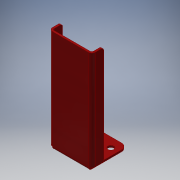
# Autodesk Inventor part: Supporto pistone pinza
Saved by Autodesk Inventor 2018 (Build 220112000, 112)
## iProperties
Created: 2020-05-29
Part Number: Supporto pistone pinza
Material: Generico
Document SubType Name: Lamiera
Designer: Francesco
Density: 1 g/cm^3
Sheet Metal Rule: Default_mm
Appearance: Rosso
Author: Francesco
Autodesk Inventor part; units mm, degrees
ref_plane "YZ Plane" through (0, 0, 0) normal (1, 0, 0) x (0, 1, 0)
ref_plane "XZ Plane" through (0, 0, 0) normal (0, 1, 0) x (-1, 0, 0)
ref_plane "XY Plane" through (0, 0, 0) normal (0, 0, 1) x (1, 0, 0)
sketch "Schizzo1" plane through (0, 0, 0) normal (0, 0, 1) x (1, 0, 0)
  line L0 (-15, 15) -> (15, 15)
  line L1 (15, 15) -> (15, -15)
  line L2 (15, -15) -> (-15, -15)
  line L3 (-15, -15) -> (-15, 15)
  line L4 (-15, 15) -> (15, -15) construction
  line L5 (15, 15) -> (-15, -15) construction
  point P0 (0, 0)
  dimension "d0" = 30
  dimension "d1" = 30
  measures "d0" distance of L1.end L2.end
  measures "d1" distance of L0.end L1.end
extrude "Piano1" add sketch "Schizzo1" along normal blind 1.5
sketch "Schizzo2" plane through (15, -16.5, 3) normal (0, -1, 0) x (1, 0, 0)
  line L0 (-30, 0) -> (0, 0)
  line L1 (0, 0) -> (0, 83.5)
  line L2 (0, 83.5) -> (-30, 83.5)
  line L3 (-30, 83.5) -> (-30, 0)
  constraints: 6 end point, 1 horizontal, 1 perpendicular, 1 vertical
edge flange "Flangia1" height 86.5 angle 90 thickness 1.5 bend radius 1.5 thickness toward (0, -1, 0) relief straight relief width 1.5 relief depth 0.75 edges at (0, -15, 1.5) wall of the first edge with corners at (-15, -16.5, 3) (15, -16.5, 3) (15, -16.5, 86.5) (-15, -16.5, 86.5)
bend "Piega (Bend)1"
corner "Angolo1"
sketch "Schizzo3" plane through (16.5, -15, 3) normal (1, 0, 0) x (0, 1, 0)
  line L0 (0, 83.5) -> (0, 0)
  line L1 (0, 0) -> (7, 0)
  line L2 (7, 0) -> (7, 83.5)
  line L3 (7, 83.5) -> (0, 83.5)
  constraints: 6 end point, 1 horizontal, 1 perpendicular, 1 vertical
edge flange "Flangia2" height 10 angle 90 thickness 1.5 bend radius 1.5 thickness toward (1, 0, 0) relief straight relief width 1.5 relief depth 0.75 corner gap 1.5 corner form 0 edges at (15, -16.5, 44.75) (-15, -16.5, 44.75) wall of the first edge with corners at (16.5, -15, 86.5) (16.5, -15, 3) (16.5, -8, 3) (16.5, -8, 86.5)
bend "Piega (Bend)2"
corner "Angolo2"
fillet "Arrotondamento angolo1" radius 5 2 edges at (-15, 15, 0.75) (15, 15, 0.75)
fillet "Arrotondamento angolo2" radius 2 4 edges at (-17.25, -8, 86.5) (-17.25, -8, 3) (17.25, -8, 86.5) (17.25, -8, 3)
sketch "Schizzo4" plane through (0, 0, 0) normal (0, 0, -1) x (-1, 0, 0)
  circle A0 centre (-9, 7) radius 3.85 projected
  circle A1 centre (9, 7) radius 3 projected
  circle A2 centre (9, -11) radius 3.6 projected
  circle A3 centre (-9, -11) radius 3 projected
  point P0 (0, 0)
  constraints: 4 coincident
hole "Foro1" at (9, 7, 0) at (-9, 7, 0) at (-9, -11, 0) at (9, -11, 0) direction (0, 0, 1) diameter 5 end through all
equation "\"d30\" = Spessore"
equation "\"d2\" = Spessore"
equation "\"d3\" = LarghezzaScaricoPiega"
equation "\"d4\" = ProfonditàScaricoPiega"
equation "\"d5\" = ResiduoMinimo"
equation "\"d6\" = RaggioTransizione"
equation "\"d9\" = RaggioPiega"
equation "\"d10\" = DimensioniScaricoAngolo"
equation "\"d11\" = DimensioneGioco"
equation "\"d12\" = Dimensione_raggio_Jacobi"
equation "\"d13\" = LarghezzaScaricoPiega"
equation "\"d14\" = ProfonditàScaricoPiega"
equation "\"d15\" = ResiduoMinimo"
equation "\"d16\" = RaggioTransizione"
equation "\"d19\" = RaggioPiega"
equation "\"d20\" = DimensioniScaricoAngolo"
equation "\"d21\" = DimensioneGioco"
equation "\"d22\" = Dimensione_raggio_Jacobi"
equation "\"RaggioPiega\" = Spessore"
equation "\"LarghezzaScaricoPiega\" = Spessore"
equation "\"ProfonditàScaricoPiega\" = 0.5 * Spessore"
equation "\"DimensioniScaricoAngolo\" = 4 * Spessore"
equation "\"ResiduoMinimo\" = 2 * Spessore"
equation "\"RaggioTransizione\" = RaggioPiega"
equation "\"Dimensione_raggio_Jacobi\" = RaggioPiega"
equation "\"DimensioneGioco\" = Spessore"
equation "\"Spessore\" = 1.5"
